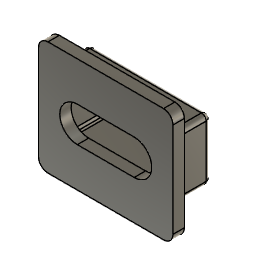
MSMD - USB Cap v6 (Autodesk Fusion 360 design; units mm, degrees)
Autodesk Fusion 360 part; units mm, degrees
sketch "Boceto1" plane through (0, 0, 0) normal (0, 1, 0) x (1, 0, 0) in component "Component"
  line L0 (-7.1, -6) -> (7.1, -6)
  line L1 (7.1, -6) -> (7.1, 6)
  line L2 (7.1, 6) -> (-7.1, 6)
  line L3 (-7.1, 6) -> (-7.1, -6)
  dimension "d1" = 7.1
  dimension "d2" = 7.1
  dimension "d3" = 6
  dimension "d4" = 6
  constraint horizontal L0
  constraint vertical L1
  constraint horizontal L2
  constraint vertical L3
  measures "d1" horizontal distance of origin L0.start
  measures "d2" horizontal distance of origin L0.end
  measures "d3" vertical distance of origin L0.start
  measures "d4" vertical distance of origin L2.end
extrude "Extruir1" add sketch "Boceto1" along normal blind 1.2 in component "Component"
fillet "Empalme1" radius 1 4 edges at (7.1, 0.6, -6) (7.1, 0.6, 6) (-7.1, 0.6, -6) (-7.1, 0.6, 6) in component "Component"
sketch "Boceto3" plane through (0, 1.2, 0) normal (0, 1, 0) x (-1, 0, 0) in component "Component"
  line L0 (-6.95, -5) -> (-6.95, -5.55)
  line L1 (3, -1.85) -> (-3, -1.85)
  line L2 (-3, -1.85) -> (-3, 1.85)
  line L3 (-3, 1.85) -> (3, 1.85)
  line L4 (3, 1.85) -> (3, -1.85)
  arc A0 (3, -1.85) -> (3, 1.85) centre (3, 0) ccw
  arc A1 (-3, 1.85) -> (-3, -1.85) centre (-3, 0) ccw
  arc A2 (7.1, 5) -> (6.1, 6) centre (6.1, 5) ccw
  line L5 (6.1, 6) -> (-6.1, 6)
  arc A3 (-6.1, 6) -> (-7.1, 5) centre (-6.1, 5) ccw
  line L6 (-7.1, 5) -> (-7.1, -5)
  arc A4 (-7.1, -5) -> (-6.1, -6) centre (-6.1, -5) ccw
  line L7 (-6.1, -6) -> (6.1, -6)
  arc A5 (6.1, -6) -> (7.1, -5) centre (6.1, -5) ccw
  line L8 (7.1, -5) -> (7.1, 5)
  point P0 (3, 0)
  point P1 (-3, 0)
  dimension "d24" = 3.7
  dimension "d25" = 6
  dimension "d26" = 3
  dimension "d27" = 1.85
  dimension "d28" = 1.85
  dimension "d77" = 6
  dimension "d80" = 12
  constraint horizontal L1
  constraint vertical L2
  constraint horizontal L3
  constraint vertical L4
  constraint coincident L4 P0
  constraint coincident P0 A0.centre
  constraint coincident L2 P1
  constraint coincident P1 A1.centre
  measures "d24" distance of L1.start L3.end
  measures "d25" distance of L1.start L1.end
  measures "d26" horizontal distance of origin L1.start
  measures "d27" distance of L1.start P0
  measures "d28" distance of L1.end P1
  measures "d77" distance of P1 L7
  measures "d80" distance of L5.end A4.end
extrude "Extruir6" cut sketch "Boceto3" against normal blind 10 contours L1 L2 L3 L4 | L4 A0 | L2 A1 in component "Component"
sketch "Boceto3 (2)" plane through (0, 1.2, 0) normal (0, 1, 0) x (-1, 0, 0)
  line L0 (-3, 1.85) -> (3, 1.85)
  arc A0 (3, -1.85) -> (3, 1.85) centre (3, 0) ccw
  line L1 (3, -1.85) -> (-3, -1.85)
  arc A1 (-3, 1.85) -> (-3, -1.85) centre (-3, 0) ccw
  arc A2 (7.1, 5) -> (6.1, 6) centre (6.1, 5) ccw
  line L2 (6.1, 6) -> (-6.1, 6)
  arc A3 (-6.1, 6) -> (-7.1, 5) centre (-6.1, 5) ccw
  line L3 (-7.1, 5) -> (-7.1, -5)
  arc A4 (-7.1, -5) -> (-6.1, -6) centre (-6.1, -5) ccw
  line L4 (-6.1, -6) -> (6.1, -6)
  arc A5 (6.1, -6) -> (7.1, -5) centre (6.1, -5) ccw
  line L5 (7.1, -5) -> (7.1, 5)
  line L6 (4.5, -1.9119) -> (-4.5, -1.9119)
  line L7 (-4.9, -1.6119) -> (-4.9, 1.9051)
  line L8 (-4.9, 1.9051) -> (4.9, 1.9051)
  line L9 (4.9, 1.9051) -> (4.9, -2.75)
  line L10 (-6.4, -3.1119) -> (-6.4, 3.4051)
  line L11 (-6.4, 3.4051) -> (6.4, 3.4051)
  line L12 (6.4, 3.4051) -> (6.4, -3.1119)
  line L13 (4.9, -2.75) -> (4.9, -3.1119)
  line L14 (-4.9, -1.6119) -> (-4.9, -3.1119)
  line L15 (4.5, -3.1119) -> (4.5, -1.9119)
  line L16 (-4.5, -3.1119) -> (-4.5, -1.9119)
  line L17 (6.4, -3.1119) -> (4.9, -3.1119)
  line L18 (4.5, -3.1119) -> (-4.5, -3.1119)
  line L19 (-4.9, -3.1119) -> (-6.4, -3.1119)
  line L20 (4.9, -3.1119) -> (4.8, -3.1119)
  line L21 (4.8, -3.1119) -> (4.8, -1.9)
  line L22 (4.8, -1.9) -> (4.9, -1.9)
  line L23 (4.9, -1.9) -> (4.9, -3.1119)
  line L24 (-4.9, -3.1119) -> (-4.8, -3.1119)
  line L25 (-4.8, -3.1119) -> (-4.8, -1.9)
  line L26 (-4.8, -1.9) -> (-4.9, -1.9)
  line L27 (-4.9, -1.9) -> (-4.9, -3.1119)
  dimension "d45" = 1.5
  dimension "d46" = 1.5
  dimension "d47" = 1.5
  dimension "d48" = 1.5
  dimension "d64" = 9.8
  dimension "d68" = 4.9
  dimension "d69" = 4.9
  dimension "d70" = 0.4
  dimension "d71" = 0.4
  dimension "d73" = 1.2
  dimension "d74" = 0.1
  dimension "d75" = 0.1
  constraint horizontal L6
  constraint vertical L7
  constraint horizontal L8
  constraint vertical L9
  constraint horizontal L17
  constraint vertical L10
  constraint horizontal L11
  constraint vertical L12
  constraint perpendicular L13 L17
  constraint coincident L14.end L17
  constraint perpendicular L14 L17
  constraint coincident L15.start L17
  constraint perpendicular L6 L15
  constraint coincident L16.start L17
  constraint perpendicular L6 L16
  constraint collinear L17 L18
  constraint collinear L18 L19
  constraint horizontal L20
  constraint vertical L21
  constraint horizontal L22
  constraint vertical L23
  constraint horizontal L24
  constraint vertical L25
  constraint horizontal L26
  constraint vertical L27
  measures "d45" horizontal distance of L8.end L11.end
  measures "d46" horizontal distance of L7.end L10.end
  measures "d47" vertical distance of L7.end L10.end
  measures "d48" vertical distance of L7.start L10.start
  measures "d64" distance of L7.end L8.end
  measures "d68" horizontal distance of origin L13.end
  measures "d69" horizontal distance of origin L7.end
  measures "d70" distance of L13.end L15.start
  measures "d71" distance of L14.end L16.start
  measures "d73" distance of L16.start L6.end
  measures "d74" distance of L13.end L20.end
  measures "d75" distance of L14.end L24.end
extrude "Extruir10" add sketch "Boceto3 (2)" along normal blind 3.5 contours L6 L15 L16 L18 | L7 L8 L9 L10 L11 L12 L13 L14 L17 L19 L23 L27 | L14 L24 L25 L26 L27 | L9 L13 L20 L21 L22 L23 in component "Component"
fillet "Empalme3" radius 0.5 24 edges at (-4.5, 2.95, -3.1119) (-4.5, 2.95, -1.9119) (4.5, 2.95, -3.1119) (4.5, 2.95, -1.9119) (-4.5, 4.7, -2.5119) (4.5, 4.7, -2.5119) (-4.9, 4.7, 0.0026) (0, 4.7, 1.9051) (4.9, 4.7, 0.0026) (-5.6, 4.7, -3.1119) (0, 4.7, -3.1119) (5.6, 4.7, -3.1119) (-6.4, 4.7, 0.1466) (0, 4.7, 3.4051) (6.4, 4.7, 0.1466) (0, 4.7, -1.9119) (-6.4, 2.95, 3.4051) (6.4, 2.95, 3.4051) (6.4, 2.95, -3.1119) (-6.4, 2.95, -3.1119) (-4.8, 2.95, -3.1119) (-4.8, 2.95, -1.9) (4.8, 2.95, -3.1119) (4.8, 2.95, -1.9) in component "Component"
component "Component" placed x (1, 0, 0) y (0, 1, 0) z (0, 0, 1) at (0, 0, 0)
equation "d2 = d1"
equation "d4 = d3"
equation "d26 = d25 / 2"
equation "d27 = d24 / 2"
equation "d28 = d27"
equation "d43 = 1.8 mm + 0.5 mm"
equation "d46 = d45"
equation "d47 = d45"
equation "d48 = d45"
equation "d71 = d70"
equation "d75 = d74"
equation "d77 = d80 / 2"
